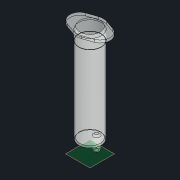
# Autodesk Inventor part: Syringe
Saved by Autodesk Inventor 2022.2 (Build 262287010, 287A)
## iProperties
Created: 2022-06-04
Part Number: Syringe
Material: Glass
Document SubType Name: Modeling
Designer: frede
Density: 2.18 g/cm^3
Appearance: Clear Reflective
Author: frede
Autodesk Inventor part; units mm, degrees
ref_plane "YZ Plane" through (0, 0, 0) normal (1, 0, 0) x (0, 1, 0)
ref_plane "XZ Plane" through (0, 0, 0) normal (0, 1, 0) x (-1, 0, 0)
ref_plane "XY Plane" through (0, 0, 0) normal (0, 0, 1) x (1, 0, 0)
sketch "Sketch1" plane through (0, 0, 0) normal (0, 1, 0) x (-1, 0, 0)
  circle A0 centre (0, 0) radius 8.575
  dimension "d0" = 17.15
  constraints: 1 centre point, 1 coincident
  measures "d0" diameter of A0
extrude "Extrusion1" add sketch "Sketch1" along normal blind 75.5
sketch "Sketch2" plane through (0, 75.5, 0) normal (0, 1, 0) x (1, 0, 0)
  circle A0 centre (0, 0) radius 8.85
  dimension "d3" = 17.7
  constraints: 1 centre point, 1 coincident
  measures "d3" diameter of A0
extrude "Extrusion2" add sketch "Sketch2" against normal blind 9.6
sketch "Sketch3" plane through (0, 75.5, 0) normal (0, 1, 0) x (1, 0, 0)
  line L0 (-3.3083, -9.5957) -> (-10.4021, -7.15)
  arc A0 (-10.4021, 7.15) -> (-10.4021, -7.15) centre (-7.937, 0) ccw
  line L1 (-10.4021, 7.15) -> (-3.3083, 9.5957)
  arc A1 (3.3083, 9.5957) -> (-3.3083, 9.5957) centre (0, 0) ccw
  line L2 (3.3083, 9.5957) -> (10.4021, 7.15)
  arc A2 (10.4021, -7.15) -> (10.4021, 7.15) centre (7.937, 0) ccw
  line L3 (10.4021, -7.15) -> (3.3083, -9.5957)
  arc A3 (-3.3083, -9.5957) -> (3.3083, -9.5957) centre (0, 0) ccw
  line L4 (0, -10.15) -> (0, 10.15) construction
  line L5 (-15.5, 0) -> (15.5, 0) construction
  dimension "d6" = 20.3
  dimension "d7" = 31
  dimension "d8" = 14.3
  constraints: 12 end point, 12 point on circle, 8 tangent, 4 centre point, 3 equal length, 2 equal radius, 2 horizontal alignment, 1 coincident
  measures "d6" distance of L4.start L4.end
  measures "d7" distance of L5.start L5.end
  measures "d8" distance of L3.start L2.end
extrude "Extrusion3" add sketch "Sketch3" against normal blind 2
sketch "Sketch4" plane through (0, 75.5, 0) normal (0, 1, 0) x (1, 0, 0)
  circle A0 centre (0, 0) radius 7.875
  dimension "d11" = 15.75
  constraints: 1 centre point, 1 coincident
  measures "d11" diameter of A0
extrude "Extrusion4" cut sketch "Sketch4" against normal blind 74.5
sketch "Sketch5" plane through (0, 0, 0) normal (0, -1, 0) x (1, 0, 0)
  circle A0 centre (0, -5.075) radius 2.5
  point P0 (0, 0)
  dimension "d14" = 5
  constraints: 1 centre point, 1 vertical alignment
  measures "d14" diameter of A0
ref_plane "Work Plane1" through (0, -10, 0) normal (0, -1, 0) x (1, 0, 0)
sketch "Sketch6" plane through (0, -10, 0) normal (0, -1, 0) x (1, 0, 0)
  circle A0 centre (0, -5.075) radius 2
  point P0 (0, 0)
  dimension "d18" = 4
  constraints: 1 centre point, 1 coincident
  measures "d18" diameter of A0
loft "Loft1" add profiles "Sketch5", "Sketch6"
sketch "Sketch7" plane through (0, -10, -5.075) normal (0, -1, 0) x (1, 0, 0)
  circle A0 centre (0, 0) radius 2 projected
  circle A1 centre (0, 0) radius 1.2
  point P0 (0, 5.075)
  dimension "d24" = 0.8
  constraints: 1 centre point
  measures "d24" radial gap between concentric circles of A0 A1
extrude "Extrusion5" cut sketch "Sketch7" against normal through all contours A1
body "Solid1"
